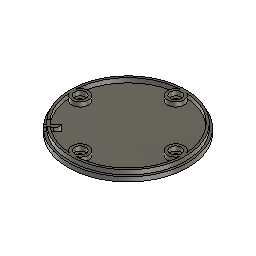
TWISTED WIFI LAMP ASSEMBLY (Autodesk Fusion 360 archive; units mm, degrees)
design "LAMP TOP COVER"
part number: 2026-05-20-23-41-38-894
Autodesk Fusion 360 part; units mm, degrees
(part 1 of 2)
sketch "Sketch1" plane through (0, 0, 0) normal (0, 0, 1) x (1, 0, 0)
  circle A0 centre (0, 0) radius 40
  circle A1 centre (0, 0) radius 38.5
  dimension "d1" = 80
  dimension "d2" = 77
  constraint coincident A0.centre A1.centre
  constraint concentric A0 A1
  measures "d1" diameter of A0
  measures "d2" diameter of A1
extrude "Extrude1" add sketch "Sketch1" along normal blind 3 contours A0 | A1
sketch "Sketch2" plane through (0, 0, 3) normal (0, 0, 1) x (-1, 0, 0)
  circle A0 centre (0, 0) radius 40
  circle A1 centre (0, 0) radius 38.5
  circle A2 centre (0, 0) radius 37
  dimension "d5" = 77
  dimension "d6" = 74
  constraint coincident A0.centre A1.centre
  constraint concentric A1 A2
  measures "d5" diameter of A1
  measures "d6" diameter of A2
extrude "Extrude2" add sketch "Sketch2" along normal blind 3 contours A1
sketch "Sketch3" plane through (0, 0, 3) normal (0, 0, 1) x (-1, 0, 0)
  circle A0 centre (0, 0) radius 37
  circle A1 centre (-32, 0) radius 5.5
  circle A2 centre (-32, 0) radius 3.75
  circle A3 centre (0, -32) radius 5.5
  circle A4 centre (0, -32) radius 3.75
  circle A5 centre (32, 0) radius 5.5
  circle A6 centre (32, 0) radius 3.75
  circle A7 centre (0, 32) radius 5.5
  circle A8 centre (0, 32) radius 3.75
  dimension "d9" = 11
  dimension "d10" = 7.5
  dimension "d11" = 32
  dimension "d13" = 360
  constraint concentric A1 A2
  measures "d9" diameter of A1
  measures "d10" diameter of A2
  measures "d11" distance of A0.centre A1.centre
extrude "Extrude3" add sketch "Sketch3" along normal blind 3 contours A0 A5 | A0 A7 | A0 A3 | A0 A1 picked at (36.1717, -2.5797) picked at (-1.5513, 36.4665) picked at (1.5513, -36.4665) picked at (-36.4974, 1.463)
sketch "Sketch4" plane through (0, 0, 3) normal (0, 0, 1) x (-1, 0, 0)
  circle A0 centre (32, 0) radius 3.75
  circle A1 centre (32, 0) radius 1.6
  circle A2 centre (0, 32) radius 1.6
  circle A3 centre (-32, 0) radius 1.6
  circle A4 centre (0, -32) radius 1.6
  dimension "d16" = 3.2
  dimension "d17" = 32
  dimension "d19" = 360
  constraint concentric A0 A1
  measures "d16" diameter of A1
  measures "d17" distance of origin A0.centre
extrude "Extrude4" cut sketch "Sketch4" against normal through all draft 25.02 contours A1 | A2 | A3 | A4
ref_plane "WorkPlane1" through (0, 0, 0) normal (-0.707107, 0.707107, 0) x (0, 0, 1)
sketch "Sketch5" plane through (0, 0, 0) normal (-0.707107, 0.707107, 0) x (0, 0, 1)
  line L0 (3, -40) -> (3, 40)
  line L1 (6, -38.5) -> (6, 38.5)
  line L2 (3, 38.5) -> (3, -38.5)
  line L3 (3, -40) -> (3, 40)
  line L4 (0, -40) -> (0, 40)
  line L5 (6, -38.5) -> (3, -38.5)
  line L6 (3, -38.5) -> (3, -36.5)
  line L7 (3, -36.5) -> (6, -36.5)
  line L8 (6, -36.5) -> (6, -38.5)
  line L9 (6, -40) -> (1, -40)
  line L10 (6, -40) -> (6, -30.653)
  line L11 (1, -40) -> (1, -35.115)
  arc A0 (6, -30.653) -> (1, -35.115) centre (5.491, -35.1151) ccw
  dimension "d21" = 2
  dimension "d22" = 3
  dimension "d23" = 5
  dimension "d24" = 3
  dimension "d25" = 9.347
  dimension "d26" = 4.885
  dimension "d27" = 4.491
  constraint horizontal L5
  constraint vertical L6
  constraint horizontal L7
  constraint vertical L8
  constraint coincident L1.start L5.start
  constraint horizontal L9
  constraint perpendicular L9 L10
  constraint perpendicular L9 L11
  constraint coincident L11.end A0.end
  measures "d21" distance of L1.start L7.end
  measures "d22" distance of L6.end L7.end
  measures "d23" distance of L9.start L9.end
  measures "d24" distance of L0 L9.start
  measures "d25" distance of L9.start L10.end
  measures "d26" distance of L9.end L11.end
  measures "d27" radius of A0
extrude "Extrude5" cut sketch "Sketch5" along normal mid plane 6

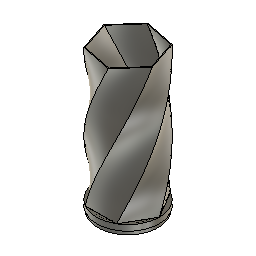
design "lamp hull"
part number: 2026-05-21-10-49-18-693
Autodesk Fusion 360 part; units mm, degrees
sketch "Sketch1" plane through (0, 0, 0) normal (0, 0, 1) x (1, 0, 0)
  circle A0 centre (0, 0) radius 38.7995
  circle A1 centre (0, 0) radius 36.9995
  dimension "d1" = 77.599
  dimension "d2" = 73.999
  constraint coincident A0.centre A1.centre
  measures "d1" diameter of A0
  measures "d2" diameter of A1
extrude "Extrude1" add sketch "Sketch1" along normal blind 4.8 from surface at 17.9
sketch "Sketch2" plane through (0, 0, 22.7) normal (0, 0, 1) x (-1, 0, 0)
  circle A0 centre (0, 0) radius 36.9995
  circle A1 centre (0, 0) radius 38.7995
  circle A2 centre (0, 0) radius 40
  dimension "d6" = 80
  constraint concentric A0 A2
  measures "d6" diameter of A2
extrude "Extrude2" add sketch "Sketch2" along normal blind 7.3 contours A1 | A2
sketch "Sketch3" plane through (0, 0, 30) normal (0, 0, 1) x (-1, 0, 0)
  circle A0 centre (0, 0) radius 36.9995
  circle A1 centre (0, 0) radius 40
  line L0 (-40, 0) -> (-20, -34.641)
  line L1 (-20, -34.641) -> (20, -34.641)
  line L2 (20, -34.641) -> (40, 0)
  line L3 (40, 0) -> (20, 34.641)
  line L4 (20, 34.641) -> (-20, 34.641)
  line L5 (-20, 34.641) -> (-40, 0)
  line L6 (38.8453, 0) -> (19.4226, 33.641)
  line L7 (19.4226, 33.641) -> (-19.4226, 33.641)
  line L8 (-19.4226, 33.641) -> (-38.8453, 0)
  line L9 (-38.8453, 0) -> (-19.4226, -33.641)
  line L10 (-19.4226, -33.641) -> (19.4226, -33.641)
  line L11 (19.4226, -33.641) -> (38.8453, 0)
  dimension "d9" = 40
  dimension "d10" = 20
  dimension "d11" = -1
  constraint coincident A0.centre A1.centre
  measures "d9" horizontal distance of L3.end L4.end
  measures "d10" horizontal distance of A0.centre L0.end
sketch "Sketch4" plane through (0, 0, 0) normal (0, 1, 0) x (1, 0, 0)
  line L0 (0, -30) -> (0, -200)
  dimension "d12" = 170
  constraint vertical L0
  measures "d12" distance of L0.start L0.end
sweep "Sweep1" add twist angle 108.3 profiles "Sketch3" path "Sketch4" along L0 section 1 contours A0 L3 L6 | A0 L2 L3 L6 L11 | A0 L2 L11 | A0 L3 L4 L6 L7 | A0 L1 L2 L10 L11 | A0 L4 L7 | A0 L1 L10 | A0 L4 L5 L7 L8 | A0 L0 L1 L9 L10 | A0 L5 L8 | A0 L0 L9 | A0 L0 L5 L8 L9
sketch "Sketch5" plane through (0, 0, 30) normal (0, 0, 1) x (-1, 0, 0)
  line L0 (-23.5007, 28.5776) -> (-20, 34.641)
  arc A0 (-20, 34.641) -> (-40, 0) centre (0, 0) ccw
  line L1 (-40, 0) -> (-36.4993, 6.0634)
  arc A1 (-23.5007, 28.5776) -> (-36.4993, 6.0634) centre (0, 0) ccw
  arc A2 (-23.5007, 28.5776) -> (-36.4993, 6.0634) centre (0, 0) ccw
  line L2 (-23.5007, 28.5776) -> (-36.4993, 6.0634)
  point P0 (-36.4993, 6.0634)
  point P1 (-23.5007, 28.5776)
extrude "Extrude3" add sketch "Sketch5" against normal blind 0.8
pattern_circular "C-Pattern1" count 6 over 360 about axis through (0, 0, 1.75) along (0, 0, 1) of "Extrude3"

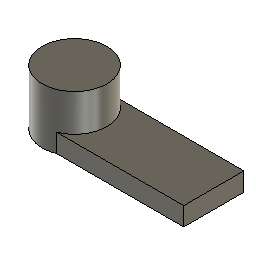
design "LAMP BUTTON"
part number: 2026-05-20-23-07-59-793
Autodesk Fusion 360 part; units mm, degrees
sketch "Sketch1" plane through (0, 0, 0) normal (0, 0, 1) x (1, 0, 0)
  circle A0 centre (0, 0) radius 3.5
  line L0 (1.299, 3.25) -> (15.041, 3.25)
  line L1 (1.299, -3.25) -> (15.041, -3.25)
  line L2 (15.041, 3.25) -> (15.041, -3.25)
  dimension "d1" = 7
  dimension "d2" = 13.742
  dimension "d3" = 13.742
  dimension "d4" = 6.5
  dimension "d5" = 3.25
  constraint coincident A0.centre origin
  constraint coincident A0 L0.start
  constraint horizontal L0
  constraint coincident A0 L1.start
  constraint horizontal L1
  measures "d1" diameter of A0
  measures "d2" distance of L1.start L1.end
  measures "d3" distance of L0.start L0.end
  measures "d4" distance of L0 L1
  measures "d5" distance of A0.centre L0
extrude "Extrude1" add sketch "Sketch1" against normal blind 6 contours A0
extrude "Extrude2" add sketch "Sketch1" along normal blind 2 from surface at -6 contours A0 L0 L1 L2

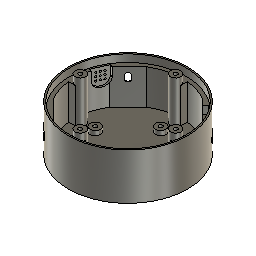
design "BOTTOM LIGHT BASE"
part number: 2026-05-20-15-01-53-421
Autodesk Fusion 360 part; units mm, degrees
sketch "Sketch1" plane through (0, 0, 0) normal (0, 0, 1) x (1, 0, 0)
  circle A0 centre (0, 0) radius 40
  circle A1 centre (0, 0) radius 39
  dimension "d1" = 80
  dimension "d2" = -1
  constraint coincident A0.centre A1.centre
  measures "d1" diameter of A0
extrude "Extrude1" add sketch "Sketch1" along normal blind 31
sketch "Sketch2" plane through (0, 0, 0) normal (0, 0, 1) x (1, 0, 0)
  circle A0 centre (0, 0) radius 39
  circle A1 centre (0, 0) radius 36.5
  dimension "d5" = 78
  dimension "d6" = 73
  constraint coincident A0.centre A1.centre
  measures "d5" diameter of A0
  measures "d6" diameter of A1
extrude "Extrude2" add sketch "Sketch2" along normal blind 2.5 contours A0 | A1
extrude "Extrude3" add sketch "Sketch2" along normal blind 23.5 from surface at 2.5
sketch "Sketch3" plane through (0, 0, 2.5) normal (0, 0, 1) x (-1, 0, 0)
  circle A0 centre (0, 0) radius 36.5
  circle A1 centre (0, 22) radius 3.5
  circle A2 centre (0, 22) radius 1.25
  circle A3 centre (-22, 0) radius 1.25
  circle A4 centre (-22, 0) radius 3.5
  circle A5 centre (0, -22) radius 1.25
  circle A6 centre (0, -22) radius 3.5
  circle A7 centre (22, 0) radius 1.25
  circle A8 centre (22, 0) radius 3.5
  dimension "d12" = 7
  dimension "d13" = 2.5
  dimension "d14" = 22
  dimension "d16" = 360
  constraint concentric A1 A2
  constraint vertical A0.centre A1.centre
  measures "d12" diameter of A1
  measures "d13" diameter of A2
  measures "d14" distance of A0.centre A1.centre
extrude "Extrude4" add sketch "Sketch3" along normal blind 3 contours A1 | A4 | A6 | A8
sketch "Sketch4" plane through (0, 0, 2.5) normal (0, 0, 1) x (-1, 0, 0)
  circle A0 centre (0, 22) radius 3.5
  circle A1 centre (-22, 0) radius 3.5
  circle A2 centre (0, 0) radius 36.5
  circle A3 centre (0, -22) radius 3.5
  circle A4 centre (22, 0) radius 3.5
  circle A5 centre (0, 32) radius 3.5
  circle A6 centre (0, 32) radius 1.25
  circle A7 centre (-32, 0) radius 3.5
  circle A8 centre (-32, 0) radius 1.25
  circle A9 centre (0, -32) radius 3.5
  circle A10 centre (0, -32) radius 1.25
  circle A11 centre (32, 0) radius 3.5
  circle A12 centre (32, 0) radius 1.25
  line L0 (3.5, 32) -> (3.5, 36.3318)
  line L1 (-3.4971, 32.1421) -> (-3.3213, 36.4703)
  line L2 (-3.5, -32) -> (-3.5, -36.3318)
  line L3 (3.5, -32) -> (3.5, -36.3318)
  line L4 (-31.9802, 3.4999) -> (-36.3294, 3.5245)
  line L5 (-31.9802, -3.4999) -> (-36.3294, -3.5245)
  line L6 (32, 3.5) -> (36.3318, 3.5)
  line L7 (32, -3.5) -> (36.3318, -3.5)
  dimension "d19" = 7
  dimension "d20" = 2.5
  dimension "d21" = 32
  dimension "d23" = 360
  constraint concentric A5 A6
  constraint vertical A2.centre A5.centre
  constraint coincident A5 L0.start
  constraint coincident A2 L0.end
  constraint vertical L0
  constraint coincident A5 L1.start
  constraint tangent A5 L1
  constraint tangent A5 L0
  constraint equal L0 L1
  constraint coincident A9 L2.start
  constraint coincident A2 L2.end
  constraint vertical L2
  constraint coincident A9 L3.start
  constraint coincident A2 L3.end
  constraint parallel L2 L3
  constraint tangent A9 L2
  constraint tangent A9 L3
  constraint coincident A7 L4.start
  constraint coincident A2 L4.end
  constraint tangent A7 L4
  constraint coincident A7 L5.start
  constraint coincident A2 L5.end
  constraint tangent A7 L5
  constraint coincident A11 L6.start
  constraint coincident A2 L6.end
  constraint horizontal L6
  constraint coincident A11 L7.start
  constraint coincident A2 L7.end
  constraint tangent A11 L7
  constraint tangent A11 L6
  constraint equal L6 L7
  constraint equal L4 L5
  measures "d19" diameter of A5
  measures "d20" diameter of A6
  measures "d21" vertical distance of A2.centre A5.centre
extrude "Extrude5" add sketch "Sketch4" along normal blind 28.5 contours A11 | A5 | A9 | A7
extrude "Extrude6" add sketch "Sketch4" along normal blind 23.5 contours A2 A11 L6 L7 | A2 A5 L0 L1 | A2 A9 L2 L3 | A2 A7 L4 L5
sketch "Sketch5" plane through (0, 0, 26) normal (0, 0, 1) x (-1, 0, 0)
  arc A0 (-36.3294, -3.5245) -> (-3.5, -36.3318) centre (0, 0) ccw
  line L0 (-36.3294, -3.5245) -> (-31.9802, -3.4999)
  arc A1 (-31.9802, 3.4999) -> (-31.9802, -3.4999) centre (-32, 0) ccw
  line L1 (-31.9802, 3.4999) -> (-36.3294, 3.5245)
  arc A2 (-3.3262, 36.3481) -> (-36.3294, 3.5245) centre (0, 0) ccw
  line L2 (-3.3262, 36.3481) -> (-3.4971, 32.1421)
  arc A3 (3.5, 32) -> (-3.4971, 32.1421) centre (0, 32) ccw
  line L3 (3.5, 32) -> (3.5, 36.3318)
  arc A4 (36.3318, 3.5) -> (3.5, 36.3318) centre (0, 0) ccw
  line L4 (36.3318, 3.5) -> (32, 3.5)
  arc A5 (32, -3.5) -> (32, 3.5) centre (32, 0) ccw
  line L5 (32, -3.5) -> (36.3318, -3.5)
  arc A6 (3.5, -36.3318) -> (36.3318, -3.5) centre (0, 0) ccw
  line L6 (3.5, -36.3318) -> (3.5, -32)
  arc A7 (-3.5, -32) -> (3.5, -32) centre (0, -32) ccw
  line L7 (-3.5, -32) -> (-3.5, -36.3318)
  circle A8 centre (0, 0) radius 39
  line L8 (18.7432, -31.32) -> (31.3167, -18.7487)
  line L9 (18.7432, 31.32) -> (31.3167, 18.7487)
  line L10 (0, 0) -> (0, -5) construction
  line L11 (-18.7432, -31.32) -> (-31.3167, -18.7487)
  dimension "d28" = 17.78
  dimension "d29" = 16.046
  dimension "d30" = 17.78
  dimension "d31" = 16.046
  dimension "d32" = 5
  constraint coincident A6 L8.start
  constraint coincident A6 L8.end
  constraint coincident A4 L9.start
  constraint coincident A4 L9.end
  constraint coincident A0.centre A2.centre
  constraint vertical L10
  constraint symmetric L8.start L10 L11.start
  constraint symmetric L8.end L10 L11.end
  measures "d28" distance of L8.start L8.end
  measures "d29" distance of A6.start L8.start
  measures "d30" distance of L9.start L9.end
  measures "d31" distance of L3.end L9.start
  measures "d32" distance of A0.centre L10.end
extrude "Extrude7" add sketch "Sketch5" against normal up to surface (23.5 mm away) contours A0 L11 | A6 L8 | A4 L9
sketch "Sketch6" plane through (-25.03, -25.0344, 0) normal (0.707045, 0.707169, 0) x (-0.707169, 0.707045, 0)
  line L0 (-8.89, 2.5) -> (8.89, 2.5)
  line L1 (8.89, 2.5) -> (8.89, 26)
  line L2 (8.89, 26) -> (-8.89, 26)
  line L3 (-8.89, 26) -> (-8.89, 2.5)
  circle A0 centre (0, 13.5) radius 4.5
  line L4 (40, 0) -> (-40, 0)
  dimension "d35" = 9
  dimension "d36" = 13.5
  measures "d35" diameter of A0
  measures "d36" distance of A0.centre L4
extrude "Extrude8" cut sketch "Sketch6" against normal blind 60 contours A0
sketch "Sketch7" plane through (-25.03, 25.0344, 0) normal (0.707045, -0.707169, 0) x (0.707169, 0.707045, 0)
  line L0 (-8.89, 2.5) -> (8.89, 2.5)
  line L1 (8.89, 2.5) -> (8.89, 26)
  line L2 (8.89, 26) -> (-8.89, 26)
  line L3 (-8.89, 26) -> (-8.89, 2.5)
  line L4 (-1.722, 21.0095) -> (-1.722, 18.9905)
  arc A0 (-1.722, 18.9905) -> (1.759, 18.9905) centre (0.0185, 18.9905) ccw
  line L5 (1.759, 18.9905) -> (1.759, 21.0095)
  arc A1 (1.759, 21.0095) -> (-1.722, 21.0095) centre (0.0185, 21.0095) ccw
  line L6 (0.0185, 21.0095) -> (0.0185, 18.9905) construction
  dimension "d39" = 5.5
  dimension "d40" = 3.481
  dimension "d41" = 14.75
  dimension "d42" = 7.131
  constraint tangent L4 A0
  constraint tangent A0 L5
  constraint parallel L4 L5
  constraint tangent L5 A1
  constraint tangent L4 A1
  constraint vertical L6
  measures "d40" distance of L4.start L5.end
  measures "d41" distance of L0 A0
  measures "d42" distance of L1 A0.end
extrude "Extrude9" cut sketch "Sketch7" against normal blind 0.698 contours L4 A0 L5 A1
extrude "Extrude10" cut sketch "Sketch7" against normal through all draft 37 from surface at -0.698 contours L4 A0 L5 A1
sketch "Sketch8" plane through (25.03, 25.0344, 0) normal (-0.707045, -0.707169, 0) x (0.707169, -0.707045, 0)
  line L0 (-8.89, 2.5) -> (8.89, 2.5)
  line L1 (8.89, 2.5) -> (8.89, 26)
  line L2 (8.89, 26) -> (-8.89, 26)
  line L3 (-8.89, 26) -> (-8.89, 2.5)
  circle A0 centre (0, 11) radius 3.75
  line L4 (40, 0) -> (-40, 0)
  line L5 (11.25, 11) -> (-3.75, 11)
  line L6 (3.75, 11) -> (3.75, 26)
  line L7 (-3.75, 11) -> (-3.75, 26)
  point P0 (3.75, 11)
  dimension "d47" = 7.5
  dimension "d48" = 11
  constraint vertical origin A0.centre
  constraint midpoint L5 P0
  constraint coincident A0 P0
  constraint coincident A0 L5.end
  constraint horizontal L5
  constraint coincident P0 L6.start
  constraint coincident L2 L6.end
  constraint perpendicular L2 L6
  constraint coincident L2 L7.end
  constraint perpendicular L2 L7
  constraint tangent A0 L7
  measures "d47" diameter of A0
  measures "d48" distance of A0.centre L4
extrude "Extrude11" cut sketch "Sketch8" against normal blind 2.6 contours L2 A0 L6 L7 | A0 L5 | A0 L5
extrude "Extrude12" cut sketch "Sketch8" against normal through all contours A0 L5 | A0 L5
sketch "Sketch9" plane through (0, 0, 26) normal (0, 0, 1) x (-1, 0, 0)
  line L0 (-29.5202, -24.2216) -> (-27.6818, -22.3829)
  line L1 (-27.6818, -22.3829) -> (-31.3167, -18.7487)
  arc A0 (-36.3294, -3.5245) -> (-31.3167, -18.7487) centre (0, 0) ccw
  line L2 (-36.3294, -3.5245) -> (-31.9802, -3.4999)
  arc A1 (-31.9802, 3.4999) -> (-31.9802, -3.4999) centre (-32, 0) ccw
  line L3 (-31.9802, 3.4999) -> (-36.3294, 3.5245)
  arc A2 (-3.3262, 36.3481) -> (-36.3294, 3.5245) centre (0, 0) ccw
  line L4 (-3.3262, 36.3481) -> (-3.4971, 32.1421)
  arc A3 (3.5, 32) -> (-3.4971, 32.1421) centre (0, 32) ccw
  line L5 (3.5, 32) -> (3.5, 36.3318)
  arc A4 (18.7432, 31.32) -> (3.5, 36.3318) centre (0, 0) ccw
  line L6 (18.7432, 31.32) -> (31.3167, 18.7487)
  arc A5 (36.3318, 3.5) -> (31.3167, 18.7487) centre (0, 0) ccw
  line L7 (36.3318, 3.5) -> (32, 3.5)
  arc A6 (32, -3.5) -> (32, 3.5) centre (32, 0) ccw
  line L8 (32, -3.5) -> (36.3318, -3.5)
  arc A7 (31.3167, -18.7487) -> (36.3318, -3.5) centre (0, 0) ccw
  line L9 (31.3167, -18.7487) -> (18.7432, -31.32)
  arc A8 (3.5, -36.3318) -> (18.7432, -31.32) centre (0, 0) ccw
  line L10 (3.5, -36.3318) -> (3.5, -32)
  arc A9 (-3.5, -32) -> (3.5, -32) centre (0, -32) ccw
  line L11 (-3.5, -32) -> (-3.5, -36.3318)
  arc A10 (-18.7432, -31.32) -> (-3.5, -36.3318) centre (0, 0) ccw
  line L12 (-18.7432, -31.32) -> (-22.3781, -27.6858)
  line L13 (-22.3781, -27.6858) -> (-24.2164, -29.5244)
  line L14 (-24.2164, -29.5244) -> (-29.5202, -24.2216)
  circle A11 centre (0, 0) radius 39
  line L15 (32.1385, -20.5117) -> (36.4457, -10.9357)
  line L16 (32.1385, -20.5117) -> (30.3555, -19.7097)
  line L17 (36.4457, -10.9357) -> (35.0184, -10.2938)
  dimension "d52" = 10.5
  dimension "d53" = 17.212
  dimension "d54" = 1.955
  dimension "d55" = 1.565
  constraint coincident L9 L16.end
  constraint perpendicular L15 L16
  constraint coincident A7 L17.end
  constraint perpendicular L15 L17
  measures "d52" distance of L15.start L15.end
  measures "d53" distance of L9.end L15.start
  measures "d54" distance of L15.start L16.end
  measures "d55" distance of L15.end L17.end
extrude "Extrude13" cut sketch "Sketch9" against normal blind 5.8 contours A7 L9 L15 L16 L17
ref_plane "WorkPlane1" through (-30.3555, 19.7097, 26) normal (0.938263, -0.345923, 0) x (0.345923, 0.938263, 0)
sketch "Sketch10" plane through (-33.1202, 12.2109, 0) normal (0.938263, -0.345923, 0) x (0.345923, 0.938263, 0)
  line L0 (7.9922, 26) -> (7.9922, 20.2)
  line L1 (7.9922, 20.2) -> (6.7581, 20.2)
  line L2 (6.7581, 20.2) -> (-2.4554, 20.2)
  line L3 (-2.4554, 20.2) -> (-2.4554, 26)
  arc A0 (-2.4554, 20.2) -> (7.9922, 20.2) centre (2.7684, 20.2) ccw
  constraint tangent L0 A0
  constraint coincident L0.end L1.start
  constraint coincident L2.end L3.start
extrude "Extrude14" cut sketch "Sketch10" along normal up to surface end surface through (-32.1385, 20.5117, 26) normal (0.911992, -0.410207, 0) offset 0
sketch "Sketch11" plane through (-34.4041, 15.4747, 0) normal (0.911992, -0.410207, 0) x (0.410207, 0.911992, 0)
  line L0 (5.523, 26) -> (-4.977, 26)
  line L1 (-4.977, 26) -> (-4.977, 20.2)
  line L2 (-4.977, 20.2) -> (-5.0858, 20.2)
  ellipse E0 centre (0.1506, 20.2) end of major axis (-5.0858, 20.2) minor radius 5.2238 (-5.0858, 20.2) -> (5.387, 20.2) ccw
  line L3 (5.387, 20.2) -> (5.523, 20.2)
  line L4 (5.523, 20.2) -> (5.523, 26)
  circle A0 centre (2.622, 23.4) radius 0.6
  circle A1 centre (0.304, 23.4) radius 0.6
  circle A2 centre (-2.014, 23.4) radius 0.6
  circle A3 centre (2.622, 20.9) radius 0.6
  circle A4 centre (0.304, 20.9) radius 0.6
  circle A5 centre (-2.014, 20.9) radius 0.6
  circle A6 centre (2.622, 18.4) radius 0.6
  circle A7 centre (0.304, 18.4) radius 0.6
  circle A8 centre (-2.014, 18.4) radius 0.6
  dimension "d60" = 1.2
  dimension "d61" = 2.6
  dimension "d62" = 2.901
  dimension "d65" = -4.636
  dimension "d66" = 0
  dimension "d69" = 0
  dimension "d70" = -5
  measures "d60" diameter of A0
  measures "d61" distance of L0 A0.centre
  measures "d62" distance of L4 A0.centre
extrude "Extrude15" cut sketch "Sketch11" against normal through all contours A0 | A1 | A2 | A3 | A4 | A5 | A6 | A7 | A8

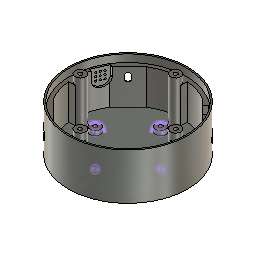
design "BOTTOM LIGHT BASE"
part number: 2026-05-20-15-01-53-421
Autodesk Fusion 360 part; units mm, degrees
sketch "Sketch1" plane through (0, 0, 0) normal (0, 0, 1) x (1, 0, 0)
  circle A0 centre (0, 0) radius 40
  circle A1 centre (0, 0) radius 39
  dimension "d1" = 80
  dimension "d2" = -1
  constraint coincident A0.centre A1.centre
  measures "d1" diameter of A0
extrude "Extrude1" add sketch "Sketch1" along normal blind 31
sketch "Sketch2" plane through (0, 0, 0) normal (0, 0, 1) x (1, 0, 0)
  circle A0 centre (0, 0) radius 39
  circle A1 centre (0, 0) radius 36.5
  dimension "d5" = 78
  dimension "d6" = 73
  constraint coincident A0.centre A1.centre
  measures "d5" diameter of A0
  measures "d6" diameter of A1
extrude "Extrude2" add sketch "Sketch2" along normal blind 2.5 contours A0 | A1
extrude "Extrude3" add sketch "Sketch2" along normal blind 23.5 from surface at 2.5
sketch "Sketch3" plane through (0, 0, 2.5) normal (0, 0, 1) x (-1, 0, 0)
  circle A0 centre (0, 0) radius 36.5
  circle A1 centre (0, 22) radius 3.5
  circle A2 centre (0, 22) radius 1.25
  circle A3 centre (-22, 0) radius 1.25
  circle A4 centre (-22, 0) radius 3.5
  circle A5 centre (0, -22) radius 1.25
  circle A6 centre (0, -22) radius 3.5
  circle A7 centre (22, 0) radius 1.25
  circle A8 centre (22, 0) radius 3.5
  dimension "d12" = 7
  dimension "d13" = 2.5
  dimension "d14" = 22
  dimension "d16" = 360
  constraint concentric A1 A2
  constraint vertical A0.centre A1.centre
  measures "d12" diameter of A1
  measures "d13" diameter of A2
  measures "d14" distance of A0.centre A1.centre
extrude "Extrude4" add sketch "Sketch3" along normal blind 3 contours A1 | A4 | A6 | A8
sketch "Sketch4" plane through (0, 0, 2.5) normal (0, 0, 1) x (-1, 0, 0)
  circle A0 centre (0, 22) radius 3.5
  circle A1 centre (-22, 0) radius 3.5
  circle A2 centre (0, 0) radius 36.5
  circle A3 centre (0, -22) radius 3.5
  circle A4 centre (22, 0) radius 3.5
  circle A5 centre (0, 32) radius 3.5
  circle A6 centre (0, 32) radius 1.25
  circle A7 centre (-32, 0) radius 3.5
  circle A8 centre (-32, 0) radius 1.25
  circle A9 centre (0, -32) radius 3.5
  circle A10 centre (0, -32) radius 1.25
  circle A11 centre (32, 0) radius 3.5
  circle A12 centre (32, 0) radius 1.25
  line L0 (3.5, 32) -> (3.5, 36.3318)
  line L1 (-3.4971, 32.1421) -> (-3.3213, 36.4703)
  line L2 (-3.5, -32) -> (-3.5, -36.3318)
  line L3 (3.5, -32) -> (3.5, -36.3318)
  line L4 (-31.9802, 3.4999) -> (-36.3294, 3.5245)
  line L5 (-31.9802, -3.4999) -> (-36.3294, -3.5245)
  line L6 (32, 3.5) -> (36.3318, 3.5)
  line L7 (32, -3.5) -> (36.3318, -3.5)
  dimension "d19" = 7
  dimension "d20" = 2.5
  dimension "d21" = 32
  dimension "d23" = 360
  constraint concentric A5 A6
  constraint vertical A2.centre A5.centre
  constraint coincident A5 L0.start
  constraint coincident A2 L0.end
  constraint vertical L0
  constraint coincident A5 L1.start
  constraint tangent A5 L1
  constraint tangent A5 L0
  constraint equal L0 L1
  constraint coincident A9 L2.start
  constraint coincident A2 L2.end
  constraint vertical L2
  constraint coincident A9 L3.start
  constraint coincident A2 L3.end
  constraint parallel L2 L3
  constraint tangent A9 L2
  constraint tangent A9 L3
  constraint coincident A7 L4.start
  constraint coincident A2 L4.end
  constraint tangent A7 L4
  constraint coincident A7 L5.start
  constraint coincident A2 L5.end
  constraint tangent A7 L5
  constraint coincident A11 L6.start
  constraint coincident A2 L6.end
  constraint horizontal L6
  constraint coincident A11 L7.start
  constraint coincident A2 L7.end
  constraint tangent A11 L7
  constraint tangent A11 L6
  constraint equal L6 L7
  constraint equal L4 L5
  measures "d19" diameter of A5
  measures "d20" diameter of A6
  measures "d21" vertical distance of A2.centre A5.centre
extrude "Extrude5" add sketch "Sketch4" along normal blind 28.5 contours A11 | A5 | A9 | A7
extrude "Extrude6" add sketch "Sketch4" along normal blind 23.5 contours A2 A11 L6 L7 | A2 A5 L0 L1 | A2 A9 L2 L3 | A2 A7 L4 L5
sketch "Sketch5" plane through (0, 0, 26) normal (0, 0, 1) x (-1, 0, 0)
  arc A0 (-36.3294, -3.5245) -> (-3.5, -36.3318) centre (0, 0) ccw
  line L0 (-36.3294, -3.5245) -> (-31.9802, -3.4999)
  arc A1 (-31.9802, 3.4999) -> (-31.9802, -3.4999) centre (-32, 0) ccw
  line L1 (-31.9802, 3.4999) -> (-36.3294, 3.5245)
  arc A2 (-3.3262, 36.3481) -> (-36.3294, 3.5245) centre (0, 0) ccw
  line L2 (-3.3262, 36.3481) -> (-3.4971, 32.1421)
  arc A3 (3.5, 32) -> (-3.4971, 32.1421) centre (0, 32) ccw
  line L3 (3.5, 32) -> (3.5, 36.3318)
  arc A4 (36.3318, 3.5) -> (3.5, 36.3318) centre (0, 0) ccw
  line L4 (36.3318, 3.5) -> (32, 3.5)
  arc A5 (32, -3.5) -> (32, 3.5) centre (32, 0) ccw
  line L5 (32, -3.5) -> (36.3318, -3.5)
  arc A6 (3.5, -36.3318) -> (36.3318, -3.5) centre (0, 0) ccw
  line L6 (3.5, -36.3318) -> (3.5, -32)
  arc A7 (-3.5, -32) -> (3.5, -32) centre (0, -32) ccw
  line L7 (-3.5, -32) -> (-3.5, -36.3318)
  circle A8 centre (0, 0) radius 39
  line L8 (18.7432, -31.32) -> (31.3167, -18.7487)
  line L9 (18.7432, 31.32) -> (31.3167, 18.7487)
  line L10 (0, 0) -> (0, -5) construction
  line L11 (-18.7432, -31.32) -> (-31.3167, -18.7487)
  dimension "d28" = 17.78
  dimension "d29" = 16.046
  dimension "d30" = 17.78
  dimension "d31" = 16.046
  dimension "d32" = 5
  constraint coincident A6 L8.start
  constraint coincident A6 L8.end
  constraint coincident A4 L9.start
  constraint coincident A4 L9.end
  constraint coincident A0.centre A2.centre
  constraint vertical L10
  constraint symmetric L8.start L10 L11.start
  constraint symmetric L8.end L10 L11.end
  measures "d28" distance of L8.start L8.end
  measures "d29" distance of A6.start L8.start
  measures "d30" distance of L9.start L9.end
  measures "d31" distance of L3.end L9.start
  measures "d32" distance of A0.centre L10.end
extrude "Extrude7" add sketch "Sketch5" against normal up to surface (23.5 mm away) contours A0 L11 | A6 L8 | A4 L9
sketch "Sketch6" plane through (-25.03, -25.0344, 0) normal (0.707045, 0.707169, 0) x (-0.707169, 0.707045, 0)
  line L0 (-8.89, 2.5) -> (8.89, 2.5)
  line L1 (8.89, 2.5) -> (8.89, 26)
  line L2 (8.89, 26) -> (-8.89, 26)
  line L3 (-8.89, 26) -> (-8.89, 2.5)
  circle A0 centre (0, 13.5) radius 4.5
  line L4 (40, 0) -> (-40, 0)
  dimension "d35" = 9
  dimension "d36" = 13.5
  measures "d35" diameter of A0
  measures "d36" distance of A0.centre L4
extrude "Extrude8" cut sketch "Sketch6" against normal blind 60 contours A0
sketch "Sketch7" plane through (-25.03, 25.0344, 0) normal (0.707045, -0.707169, 0) x (0.707169, 0.707045, 0)
  line L0 (-8.89, 2.5) -> (8.89, 2.5)
  line L1 (8.89, 2.5) -> (8.89, 26)
  line L2 (8.89, 26) -> (-8.89, 26)
  line L3 (-8.89, 26) -> (-8.89, 2.5)
  line L4 (-1.722, 21.0095) -> (-1.722, 18.9905)
  arc A0 (-1.722, 18.9905) -> (1.759, 18.9905) centre (0.0185, 18.9905) ccw
  line L5 (1.759, 18.9905) -> (1.759, 21.0095)
  arc A1 (1.759, 21.0095) -> (-1.722, 21.0095) centre (0.0185, 21.0095) ccw
  line L6 (0.0185, 21.0095) -> (0.0185, 18.9905) construction
  dimension "d39" = 5.5
  dimension "d40" = 3.481
  dimension "d41" = 14.75
  dimension "d42" = 7.131
  constraint tangent L4 A0
  constraint tangent A0 L5
  constraint parallel L4 L5
  constraint tangent L5 A1
  constraint tangent L4 A1
  constraint vertical L6
  measures "d40" distance of L4.start L5.end
  measures "d41" distance of L0 A0
  measures "d42" distance of L1 A0.end
extrude "Extrude9" cut sketch "Sketch7" against normal blind 0.698 contours L4 A0 L5 A1
extrude "Extrude10" cut sketch "Sketch7" against normal through all draft 37 from surface at -0.698 contours L4 A0 L5 A1
sketch "Sketch8" plane through (25.03, 25.0344, 0) normal (-0.707045, -0.707169, 0) x (0.707169, -0.707045, 0)
  line L0 (-8.89, 2.5) -> (8.89, 2.5)
  line L1 (8.89, 2.5) -> (8.89, 26)
  line L2 (8.89, 26) -> (-8.89, 26)
  line L3 (-8.89, 26) -> (-8.89, 2.5)
  circle A0 centre (0, 11) radius 3.75
  line L4 (40, 0) -> (-40, 0)
  line L5 (11.25, 11) -> (-3.75, 11)
  line L6 (3.75, 11) -> (3.75, 26)
  line L7 (-3.75, 11) -> (-3.75, 26)
  point P0 (3.75, 11)
  dimension "d47" = 7.5
  dimension "d48" = 11
  constraint vertical origin A0.centre
  constraint midpoint L5 P0
  constraint coincident A0 P0
  constraint coincident A0 L5.end
  constraint horizontal L5
  constraint coincident P0 L6.start
  constraint coincident L2 L6.end
  constraint perpendicular L2 L6
  constraint coincident L2 L7.end
  constraint perpendicular L2 L7
  constraint tangent A0 L7
  measures "d47" diameter of A0
  measures "d48" distance of A0.centre L4
extrude "Extrude11" cut sketch "Sketch8" against normal blind 2.6 contours L2 A0 L6 L7 | A0 L5 | A0 L5
extrude "Extrude12" cut sketch "Sketch8" against normal through all contours A0 L5 | A0 L5
sketch "Sketch9" plane through (0, 0, 26) normal (0, 0, 1) x (-1, 0, 0)
  line L0 (-29.5202, -24.2216) -> (-27.6818, -22.3829)
  line L1 (-27.6818, -22.3829) -> (-31.3167, -18.7487)
  arc A0 (-36.3294, -3.5245) -> (-31.3167, -18.7487) centre (0, 0) ccw
  line L2 (-36.3294, -3.5245) -> (-31.9802, -3.4999)
  arc A1 (-31.9802, 3.4999) -> (-31.9802, -3.4999) centre (-32, 0) ccw
  line L3 (-31.9802, 3.4999) -> (-36.3294, 3.5245)
  arc A2 (-3.3262, 36.3481) -> (-36.3294, 3.5245) centre (0, 0) ccw
  line L4 (-3.3262, 36.3481) -> (-3.4971, 32.1421)
  arc A3 (3.5, 32) -> (-3.4971, 32.1421) centre (0, 32) ccw
  line L5 (3.5, 32) -> (3.5, 36.3318)
  arc A4 (18.7432, 31.32) -> (3.5, 36.3318) centre (0, 0) ccw
  line L6 (18.7432, 31.32) -> (31.3167, 18.7487)
  arc A5 (36.3318, 3.5) -> (31.3167, 18.7487) centre (0, 0) ccw
  line L7 (36.3318, 3.5) -> (32, 3.5)
  arc A6 (32, -3.5) -> (32, 3.5) centre (32, 0) ccw
  line L8 (32, -3.5) -> (36.3318, -3.5)
  arc A7 (31.3167, -18.7487) -> (36.3318, -3.5) centre (0, 0) ccw
  line L9 (31.3167, -18.7487) -> (18.7432, -31.32)
  arc A8 (3.5, -36.3318) -> (18.7432, -31.32) centre (0, 0) ccw
  line L10 (3.5, -36.3318) -> (3.5, -32)
  arc A9 (-3.5, -32) -> (3.5, -32) centre (0, -32) ccw
  line L11 (-3.5, -32) -> (-3.5, -36.3318)
  arc A10 (-18.7432, -31.32) -> (-3.5, -36.3318) centre (0, 0) ccw
  line L12 (-18.7432, -31.32) -> (-22.3781, -27.6858)
  line L13 (-22.3781, -27.6858) -> (-24.2164, -29.5244)
  line L14 (-24.2164, -29.5244) -> (-29.5202, -24.2216)
  circle A11 centre (0, 0) radius 39
  line L15 (32.1385, -20.5117) -> (36.4457, -10.9357)
  line L16 (32.1385, -20.5117) -> (30.3555, -19.7097)
  line L17 (36.4457, -10.9357) -> (35.0184, -10.2938)
  dimension "d52" = 10.5
  dimension "d53" = 17.212
  dimension "d54" = 1.955
  dimension "d55" = 1.565
  constraint coincident L9 L16.end
  constraint perpendicular L15 L16
  constraint coincident A7 L17.end
  constraint perpendicular L15 L17
  measures "d52" distance of L15.start L15.end
  measures "d53" distance of L9.end L15.start
  measures "d54" distance of L15.start L16.end
  measures "d55" distance of L15.end L17.end
extrude "Extrude13" cut sketch "Sketch9" against normal blind 5.8 contours A7 L9 L15 L16 L17
ref_plane "WorkPlane1" through (-30.3555, 19.7097, 26) normal (0.938263, -0.345923, 0) x (0.345923, 0.938263, 0)
sketch "Sketch10" plane through (-33.1202, 12.2109, 0) normal (0.938263, -0.345923, 0) x (0.345923, 0.938263, 0)
  line L0 (7.9922, 26) -> (7.9922, 20.2)
  line L1 (7.9922, 20.2) -> (6.7581, 20.2)
  line L2 (6.7581, 20.2) -> (-2.4554, 20.2)
  line L3 (-2.4554, 20.2) -> (-2.4554, 26)
  arc A0 (-2.4554, 20.2) -> (7.9922, 20.2) centre (2.7684, 20.2) ccw
  constraint tangent L0 A0
  constraint coincident L0.end L1.start
  constraint coincident L2.end L3.start
extrude "Extrude14" cut sketch "Sketch10" along normal up to surface end surface through (-32.1385, 20.5117, 26) normal (0.911992, -0.410207, 0) offset 0
sketch "Sketch11" plane through (-34.4041, 15.4747, 0) normal (0.911992, -0.410207, 0) x (0.410207, 0.911992, 0)
  line L0 (5.523, 26) -> (-4.977, 26)
  line L1 (-4.977, 26) -> (-4.977, 20.2)
  line L2 (-4.977, 20.2) -> (-5.0858, 20.2)
  ellipse E0 centre (0.1506, 20.2) end of major axis (-5.0858, 20.2) minor radius 5.2238 (-5.0858, 20.2) -> (5.387, 20.2) ccw
  line L3 (5.387, 20.2) -> (5.523, 20.2)
  line L4 (5.523, 20.2) -> (5.523, 26)
  circle A0 centre (2.622, 23.4) radius 0.6
  circle A1 centre (0.304, 23.4) radius 0.6
  circle A2 centre (-2.014, 23.4) radius 0.6
  circle A3 centre (2.622, 20.9) radius 0.6
  circle A4 centre (0.304, 20.9) radius 0.6
  circle A5 centre (-2.014, 20.9) radius 0.6
  circle A6 centre (2.622, 18.4) radius 0.6
  circle A7 centre (0.304, 18.4) radius 0.6
  circle A8 centre (-2.014, 18.4) radius 0.6
  dimension "d60" = 1.2
  dimension "d61" = 2.6
  dimension "d62" = 2.901
  dimension "d65" = -4.636
  dimension "d66" = 0
  dimension "d69" = 0
  dimension "d70" = -5
  measures "d60" diameter of A0
  measures "d61" distance of L0 A0.centre
  measures "d62" distance of L4 A0.centre
extrude "Extrude15" cut sketch "Sketch11" against normal through all contours A0 | A1 | A2 | A3 | A4 | A5 | A6 | A7 | A8
sketch "Sketch12" plane through (0, 0, 2.5) normal (0, 0, 1) x (-1, 0, 0)
  line L0 (31.3167, 18.7487) -> (18.7432, 31.32)
  arc A0 (18.7432, 31.32) -> (3.5, 36.3318) centre (0, 0) ccw
  line L1 (3.5, 36.3318) -> (3.5, 32)
  arc A1 (-3.4971, 32.1421) -> (3.5, 32) centre (0, 32) ccw
  line L2 (-3.4971, 32.1421) -> (-3.3262, 36.3481)
  arc A2 (-3.3262, 36.3481) -> (-36.3294, 3.5245) centre (0, 0) ccw
  line L3 (-36.3294, 3.5245) -> (-31.9802, 3.4999)
  arc A3 (-31.9802, -3.4999) -> (-31.9802, 3.4999) centre (-32, 0) ccw
  line L4 (-31.9802, -3.4999) -> (-36.3294, -3.5245)
  arc A4 (-36.3294, -3.5245) -> (-31.3167, -18.7487) centre (0, 0) ccw
  line L5 (-31.3167, -18.7487) -> (-18.7432, -31.32)
  arc A5 (-18.7432, -31.32) -> (-3.5, -36.3318) centre (0, 0) ccw
  line L6 (-3.5, -36.3318) -> (-3.5, -32)
  arc A6 (3.5, -32) -> (-3.5, -32) centre (0, -32) ccw
  line L7 (3.5, -32) -> (3.5, -36.3318)
  arc A7 (3.5, -36.3318) -> (18.7432, -31.32) centre (0, 0) ccw
  line L8 (18.7432, -31.32) -> (31.3167, -18.7487)
  arc A8 (31.3167, -18.7487) -> (36.3318, -3.5) centre (0, 0) ccw
  line L9 (36.3318, -3.5) -> (32, -3.5)
  arc A9 (32, 3.5) -> (32, -3.5) centre (32, 0) ccw
  line L10 (32, 3.5) -> (36.3318, 3.5)
  arc A10 (36.3318, 3.5) -> (31.3167, 18.7487) centre (0, 0) ccw
  circle A11 centre (0, 22) radius 3.5
  circle A12 centre (-22, 0) radius 3.5
  circle A13 centre (0, -22) radius 3.5
  circle A14 centre (22, 0) radius 3.5
  circle A15 centre (0, -22) radius 1.25
  circle A16 centre (-22, 0) radius 1.25
  circle A17 centre (22, 0) radius 1.25
  circle A18 centre (0, 22) radius 1.25

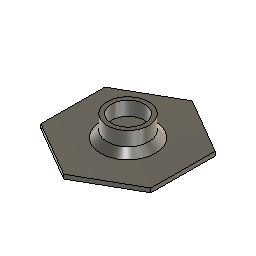
design "LAMP TWISTED TOP"
part number: 2026-05-21-08-55-42-044
Autodesk Fusion 360 part; units mm, degrees
sketch "Sketch1" plane through (0, 0, 0) normal (0, 0, 1) x (1, 0, 0)
  line L0 (33.3191, -19.4816) -> (33.5311, 19.1144)
  line L1 (33.5311, 19.1144) -> (0.212, 38.596)
  line L2 (0.212, 38.596) -> (-33.3191, 19.4816)
  line L3 (-33.3191, 19.4816) -> (-33.5311, -19.1144)
  line L4 (-33.5311, -19.1144) -> (-0.212, -38.596)
  line L5 (-0.212, -38.596) -> (33.3191, -19.4816)
  dimension "d11" = 38.596
  measures "d11" vertical distance of L4.end origin
extrude "Extrude1" add sketch "Sketch1" along normal blind 2.5
sketch "Sketch2" plane through (0, 0, 2.5) normal (0, 0, 1) x (-1, 0, 0)
  line L0 (0.212, 38.596) -> (-33.3191, 19.4816)
  line L1 (-33.3191, 19.4816) -> (-33.5311, -19.1144)
  line L2 (-33.5311, -19.1144) -> (-0.212, -38.596)
  line L3 (-0.212, -38.596) -> (33.3191, -19.4816)
  line L4 (33.3191, -19.4816) -> (33.5311, 19.1144)
  line L5 (33.5311, 19.1144) -> (0.212, 38.596)
  circle A0 centre (0, 0) radius 16.5
  dimension "d4" = 33
  constraint coincident A0.centre origin
  measures "d4" diameter of A0
extrude "Extrude2" add sketch "Sketch2" along normal blind 4 draft -45 contours A0
sketch "Sketch3" plane through (0, 0, 6.5) normal (0, 0, 1) x (-1, 0, 0)
  circle A0 centre (0, 0) radius 12.5
  circle A1 centre (0, 0) radius 12.5
  circle A2 centre (0, 0) radius 10
  dimension "d7" = 25
  dimension "d8" = 20
  constraint coincident A0.centre A1.centre
  constraint concentric A1 A2
  measures "d7" diameter of A1
  measures "d8" diameter of A2
extrude "Extrude3" add sketch "Sketch3" along normal blind 8.5

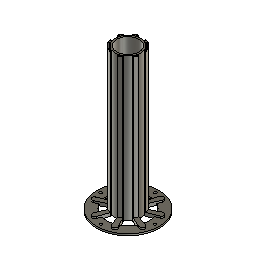
design "LAMP CORE"
part number: 2026-05-21-09-26-11-656
Autodesk Fusion 360 part; units mm, degrees
sketch "Sketch1" plane through (0, 0, 0) normal (0, 0, 1) x (1, 0, 0)
  circle A0 centre (0, 0) radius 36.6
  circle A1 centre (0, 0) radius 25
  dimension "d1" = 73.2
  dimension "d2" = 50
  constraint coincident A0.centre A1.centre
  constraint concentric A0 A1
  measures "d1" diameter of A0
  measures "d2" diameter of A1
extrude "Extrude1" add sketch "Sketch1" along normal blind 2 makes body 1
sketch "Sketch2" plane through (0, 0, 0) normal (0, 0, 1) x (1, 0, 0)
  circle A0 centre (0, 0) radius 15
  circle A1 centre (0, 0) radius 13
  dimension "d5" = 30
  dimension "d6" = 26
  constraint coincident A0.centre A1.centre
  constraint concentric A0 A1
  measures "d5" diameter of A0
  measures "d6" diameter of A1
extrude "Extrude2" add sketch "Sketch2" along normal blind 168 separate body makes body 2
sketch "Sketch3" plane through (0, 0, 168) normal (0, 0, 1) x (-1, 0, 0)
  circle A0 centre (0, 0) radius 13
  circle A1 centre (0, 0) radius 15
  line L0 (6.4849, 13.5258) -> (6.9618, 14.6269)
  line L1 (4.978, 14.1499) -> (5.3635, 15.2863)
  line L2 (5.3635, 15.2863) -> (3.943, 15.7682)
  line L3 (6.9618, 14.6269) -> (8.3382, 14.0307)
  line L4 (8.3382, 14.0307) -> (8.7357, 14.9483)
  line L5 (3.943, 15.7682) -> (4.2642, 16.7152)
  arc A2 (8.7357, 14.9483) -> (4.2642, 16.7152) centre (0.2494, 0.0129) ccw
  line L6 (-6.4855, 13.5255) -> (-7.0165, 14.6016)
  line L7 (-7.0165, 14.6016) -> (-8.3616, 13.9379)
  line L8 (-8.3616, 13.9379) -> (-8.8041, 14.8347)
  arc A3 (-4.393, 16.7471) -> (-8.8041, 14.8347) centre (0.1672, 0.1855) ccw
  line L9 (-4.0252, 15.8172) -> (-4.393, 16.7471)
  line L10 (-5.42, 15.2655) -> (-4.0252, 15.8172)
  line L11 (-4.9787, 14.1497) -> (-5.42, 15.2655)
  line L12 (-14.1499, 4.978) -> (-15.2863, 5.3635)
  line L13 (-15.2863, 5.3635) -> (-15.7682, 3.943)
  line L14 (-15.7682, 3.943) -> (-16.7152, 4.2642)
  arc A4 (-14.9483, 8.7357) -> (-16.7152, 4.2642) centre (-0.0129, 0.2494) ccw
  line L15 (-14.0307, 8.3382) -> (-14.9483, 8.7357)
  line L16 (-14.6269, 6.9618) -> (-14.0307, 8.3382)
  line L17 (-13.5258, 6.4849) -> (-14.6269, 6.9618)
  line L18 (-13.5255, -6.4855) -> (-14.6016, -7.0165)
  line L19 (-14.6016, -7.0165) -> (-13.9379, -8.3616)
  line L20 (-13.9379, -8.3616) -> (-14.8347, -8.8041)
  arc A5 (-16.7471, -4.393) -> (-14.8347, -8.8041) centre (-0.1855, 0.1672) ccw
  line L21 (-15.8172, -4.0252) -> (-16.7471, -4.393)
  line L22 (-15.2655, -5.42) -> (-15.8172, -4.0252)
  line L23 (-14.1497, -4.9787) -> (-15.2655, -5.42)
  line L24 (-4.978, -14.1499) -> (-5.3635, -15.2863)
  line L25 (-5.3635, -15.2863) -> (-3.943, -15.7682)
  line L26 (-3.943, -15.7682) -> (-4.2642, -16.7152)
  arc A6 (-8.7357, -14.9483) -> (-4.2642, -16.7152) centre (-0.2494, -0.0129) ccw
  line L27 (-8.3382, -14.0307) -> (-8.7357, -14.9483)
  line L28 (-6.9618, -14.6269) -> (-8.3382, -14.0307)
  line L29 (-6.4849, -13.5258) -> (-6.9618, -14.6269)
  line L30 (6.4855, -13.5255) -> (7.0165, -14.6016)
  line L31 (7.0165, -14.6016) -> (8.3616, -13.9379)
  line L32 (8.3616, -13.9379) -> (8.8041, -14.8347)
  arc A7 (4.393, -16.7471) -> (8.8041, -14.8347) centre (-0.1672, -0.1855) ccw
  line L33 (4.0252, -15.8172) -> (4.393, -16.7471)
  line L34 (5.42, -15.2655) -> (4.0252, -15.8172)
  line L35 (4.9787, -14.1497) -> (5.42, -15.2655)
  line L36 (14.1499, -4.978) -> (15.2863, -5.3635)
  line L37 (15.2863, -5.3635) -> (15.7682, -3.943)
  line L38 (15.7682, -3.943) -> (16.7152, -4.2642)
  arc A8 (14.9483, -8.7357) -> (16.7152, -4.2642) centre (0.0129, -0.2494) ccw
  line L39 (14.0307, -8.3382) -> (14.9483, -8.7357)
  line L40 (14.6269, -6.9618) -> (14.0307, -8.3382)
  line L41 (13.5258, -6.4849) -> (14.6269, -6.9618)
  line L42 (13.5255, 6.4855) -> (14.6016, 7.0165)
  line L43 (14.6016, 7.0165) -> (13.9379, 8.3616)
  line L44 (13.9379, 8.3616) -> (14.8347, 8.8041)
  arc A9 (16.7471, 4.393) -> (14.8347, 8.8041) centre (0.1855, -0.1672) ccw
  line L45 (15.8172, 4.0252) -> (16.7471, 4.393)
  line L46 (15.2655, 5.42) -> (15.8172, 4.0252)
  line L47 (14.1497, 4.9787) -> (15.2655, 5.42)
  dimension "d9" = 1.729
  dimension "d10" = 4.978
  dimension "d11" = 1.2
  dimension "d12" = 1.2
  dimension "d13" = 1.5
  dimension "d14" = 1.5
  dimension "d15" = 3.943
  dimension "d16" = 1
  dimension "d17" = 1
  dimension "d18" = 17.178
  dimension "d19" = 1.631
  dimension "d21" = 360
  constraint coincident A1 L0.start
  constraint coincident A1 L1.start
  constraint perpendicular L1 L2
  constraint perpendicular L0 L3
  constraint perpendicular L3 L4
  constraint perpendicular L2 L5
  measures "d9" distance of L0.end L1.end
  measures "d10" horizontal distance of A0.centre L1.start
  measures "d11" distance of L1.start L1.end
  measures "d12" distance of L0.start L0.end
  measures "d13" distance of L1.end L2.end
  measures "d14" distance of L0.end L3.end
  measures "d15" horizontal distance of A0.centre L2.end
  measures "d16" distance of L2.end L5.end
  measures "d17" distance of L3.end L4.end
  measures "d18" radius of A2
  measures "d19" distance of L0.start L1.start
extrude "Extrude3" add sketch "Sketch3" against normal blind 168 contours A1 L42 L43 L44 A9 L45 L46 L47 | A1 L36 L37 L38 A8 L39 L40 L41 | A1 L0 L1 L2 L3 L4 L5 A2 | A1 L30 L31 L32 A7 L33 L34 L35 | A1 L6 L7 L8 A3 L9 L10 L11 | A1 L24 L25 L26 A6 L27 L28 L29 | A1 L12 L13 L14 A4 L15 L16 L17 | A1 L18 L19 L20 A5 L21 L22 L23 bodies 2
sketch "Sketch4" plane through (0, 0, 0) normal (0, 0, 1) x (1, 0, 0)
  circle A0 centre (0, 0) radius 13
  arc A1 (-4.978, -14.1499) -> (4.9787, -14.1497) centre (0, 0) ccw
  line L0 (4.9787, -14.1497) -> (5.42, -15.2655)
  line L1 (5.42, -15.2655) -> (4.0252, -15.8172)
  line L2 (4.0252, -15.8172) -> (4.393, -16.7471)
  arc A2 (4.393, -16.7471) -> (8.8041, -14.8347) centre (-0.1672, -0.1855) ccw
  line L3 (8.8041, -14.8347) -> (8.3616, -13.9379)
  line L4 (8.3616, -13.9379) -> (7.0165, -14.6016)
  line L5 (7.0165, -14.6016) -> (6.4855, -13.5255)
  arc A3 (6.4855, -13.5255) -> (13.5258, -6.4849) centre (0, 0) ccw
  line L6 (13.5258, -6.4849) -> (14.6269, -6.9618)
  line L7 (14.6269, -6.9618) -> (14.0307, -8.3382)
  line L8 (14.0307, -8.3382) -> (14.9483, -8.7357)
  arc A4 (14.9483, -8.7357) -> (16.7152, -4.2642) centre (0.0129, -0.2494) ccw
  line L9 (16.7152, -4.2642) -> (15.7682, -3.943)
  line L10 (15.7682, -3.943) -> (15.2863, -5.3635)
  line L11 (15.2863, -5.3635) -> (14.1499, -4.978)
  arc A5 (14.1499, -4.978) -> (14.1497, 4.9787) centre (0, 0) ccw
  line L12 (14.1497, 4.9787) -> (15.2655, 5.42)
  line L13 (15.2655, 5.42) -> (15.8172, 4.0252)
  line L14 (15.8172, 4.0252) -> (16.7471, 4.393)
  arc A6 (16.7471, 4.393) -> (14.8347, 8.8041) centre (0.1855, -0.1672) ccw
  line L15 (14.8347, 8.8041) -> (13.9379, 8.3616)
  line L16 (13.9379, 8.3616) -> (14.6016, 7.0165)
  line L17 (14.6016, 7.0165) -> (13.5255, 6.4855)
  arc A7 (13.5255, 6.4855) -> (6.4849, 13.5258) centre (0, 0) ccw
  line L18 (6.4849, 13.5258) -> (6.9618, 14.6269)
  line L19 (6.9618, 14.6269) -> (8.3382, 14.0307)
  line L20 (8.3382, 14.0307) -> (8.7357, 14.9483)
  arc A8 (8.7357, 14.9483) -> (4.2642, 16.7152) centre (0.2494, 0.0129) ccw
  line L21 (4.2642, 16.7152) -> (3.943, 15.7682)
  line L22 (3.943, 15.7682) -> (5.3635, 15.2863)
  line L23 (5.3635, 15.2863) -> (4.978, 14.1499)
  arc A9 (4.978, 14.1499) -> (-4.9787, 14.1497) centre (0, 0) ccw
  line L24 (-4.9787, 14.1497) -> (-5.42, 15.2655)
  line L25 (-5.42, 15.2655) -> (-4.0252, 15.8172)
  line L26 (-4.0252, 15.8172) -> (-4.393, 16.7471)
  arc A10 (-4.393, 16.7471) -> (-8.8041, 14.8347) centre (0.1672, 0.1855) ccw
  line L27 (-8.8041, 14.8347) -> (-8.3616, 13.9379)
  line L28 (-8.3616, 13.9379) -> (-7.0165, 14.6016)
  line L29 (-7.0165, 14.6016) -> (-6.4855, 13.5255)
  arc A11 (-6.4855, 13.5255) -> (-13.5258, 6.4849) centre (0, 0) ccw
  line L30 (-13.5258, 6.4849) -> (-14.6269, 6.9618)
  line L31 (-14.6269, 6.9618) -> (-14.0307, 8.3382)
  line L32 (-14.0307, 8.3382) -> (-14.9483, 8.7357)
  arc A12 (-14.9483, 8.7357) -> (-16.7152, 4.2642) centre (-0.0129, 0.2494) ccw
  line L33 (-16.7152, 4.2642) -> (-15.7682, 3.943)
  line L34 (-15.7682, 3.943) -> (-15.2863, 5.3635)
  line L35 (-15.2863, 5.3635) -> (-14.1499, 4.978)
  arc A13 (-14.1499, 4.978) -> (-14.1497, -4.9787) centre (0, 0) ccw
  line L36 (-14.1497, -4.9787) -> (-15.2655, -5.42)
  line L37 (-15.2655, -5.42) -> (-15.8172, -4.0252)
  line L38 (-15.8172, -4.0252) -> (-16.7471, -4.393)
  arc A14 (-16.7471, -4.393) -> (-14.8347, -8.8041) centre (-0.1855, 0.1672) ccw
  line L39 (-14.8347, -8.8041) -> (-13.9379, -8.3616)
  line L40 (-13.9379, -8.3616) -> (-14.6016, -7.0165)
  line L41 (-14.6016, -7.0165) -> (-13.5255, -6.4855)
  arc A15 (-13.5255, -6.4855) -> (-6.4849, -13.5258) centre (0, 0) ccw
  line L42 (-6.4849, -13.5258) -> (-6.9618, -14.6269)
  line L43 (-6.9618, -14.6269) -> (-8.3382, -14.0307)
  line L44 (-8.3382, -14.0307) -> (-8.7357, -14.9483)
  arc A16 (-8.7357, -14.9483) -> (-4.2642, -16.7152) centre (-0.2494, -0.0129) ccw
  line L45 (-4.2642, -16.7152) -> (-3.943, -15.7682)
  line L46 (-3.943, -15.7682) -> (-5.3635, -15.2863)
  line L47 (-5.3635, -15.2863) -> (-4.978, -14.1499)
  line L48 (14.8347, 8.8041) -> (26.2662, 14.5848)
  line L49 (16.7471, 4.393) -> (28.6592, 9.1045)
  arc A17 (28.6592, 9.1045) -> (26.2662, 14.5848) centre (27.4627, 11.8446) ccw
  line L50 (14.8347, 8.8041) -> (13.9379, 8.3616)
  line L51 (14.8347, 8.8041) -> (13.9379, 8.3616)
  line L52 (15.8172, 4.0252) -> (16.7471, 4.393)
  line L53 (13.9379, 8.3616) -> (15.8172, 4.0252)
  line L54 (8.7357, 14.9483) -> (13.8273, 26.703)
  arc A18 (13.8273, 26.703) -> (8.26, 28.886) centre (11.0437, 27.7945) ccw
  line L55 (4.2642, 16.7152) -> (8.26, 28.886)
  line L56 (4.2642, 16.7152) -> (3.943, 15.7682)
  line L57 (3.943, 15.7682) -> (8.3382, 14.0307)
  line L58 (8.3382, 14.0307) -> (8.7357, 14.9483)
  line L59 (-4.393, 16.7471) -> (-9.1045, 28.6592)
  arc A19 (-9.1045, 28.6592) -> (-14.5848, 26.2662) centre (-11.8446, 27.4627) ccw
  line L60 (-8.8041, 14.8347) -> (-14.5848, 26.2662)
  line L61 (-8.8041, 14.8347) -> (-8.3616, 13.9379)
  line L62 (-8.3616, 13.9379) -> (-4.0252, 15.8172)
  line L63 (-4.0252, 15.8172) -> (-4.393, 16.7471)
  line L64 (-14.9483, 8.7357) -> (-26.703, 13.8273)
  arc A20 (-26.703, 13.8273) -> (-28.886, 8.26) centre (-27.7945, 11.0437) ccw
  line L65 (-16.7152, 4.2642) -> (-28.886, 8.26)
  line L66 (-16.7152, 4.2642) -> (-15.7682, 3.943)
  line L67 (-15.7682, 3.943) -> (-14.0307, 8.3382)
  line L68 (-14.0307, 8.3382) -> (-14.9483, 8.7357)
  line L69 (-16.7471, -4.393) -> (-28.6592, -9.1045)
  arc A21 (-28.6592, -9.1045) -> (-26.2662, -14.5848) centre (-27.4627, -11.8446) ccw
  line L70 (-14.8347, -8.8041) -> (-26.2662, -14.5848)
  line L71 (-14.8347, -8.8041) -> (-13.9379, -8.3616)
  line L72 (-13.9379, -8.3616) -> (-15.8172, -4.0252)
  line L73 (-15.8172, -4.0252) -> (-16.7471, -4.393)
  line L74 (-8.7357, -14.9483) -> (-13.8273, -26.703)
  arc A22 (-13.8273, -26.703) -> (-8.26, -28.886) centre (-11.0437, -27.7945) ccw
  line L75 (-4.2642, -16.7152) -> (-8.26, -28.886)
  line L76 (-4.2642, -16.7152) -> (-3.943, -15.7682)
  line L77 (-3.943, -15.7682) -> (-8.3382, -14.0307)
  line L78 (-8.3382, -14.0307) -> (-8.7357, -14.9483)
  line L79 (4.393, -16.7471) -> (9.1045, -28.6592)
  arc A23 (9.1045, -28.6592) -> (14.5848, -26.2662) centre (11.8446, -27.4627) ccw
  line L80 (8.8041, -14.8347) -> (14.5848, -26.2662)
  line L81 (8.8041, -14.8347) -> (8.3616, -13.9379)
  line L82 (8.3616, -13.9379) -> (4.0252, -15.8172)
  line L83 (4.0252, -15.8172) -> (4.393, -16.7471)
  line L84 (14.9483, -8.7357) -> (26.703, -13.8273)
  arc A24 (26.703, -13.8273) -> (28.886, -8.26) centre (27.7945, -11.0437) ccw
  line L85 (16.7152, -4.2642) -> (28.886, -8.26)
  line L86 (16.7152, -4.2642) -> (15.7682, -3.943)
  line L87 (15.7682, -3.943) -> (14.0307, -8.3382)
  line L88 (14.0307, -8.3382) -> (14.9483, -8.7357)
  dimension "d24" = 5.98
  dimension "d25" = 12.81
  dimension "d27" = 2.99
  dimension "d28" = 12.81
  dimension "d30" = 360
  constraint coincident A6.end L15.start
  constraint coincident L14.end A6.start
  constraint perpendicular L13 L49
  constraint coincident L15.end L16.start
  constraint coincident L13.end L14.start
  measures "d24" distance of L48.end L49.end
  measures "d25" distance of L14.end L49.end
  measures "d27" radius of A17
  measures "d28" distance of A6.end L48.end